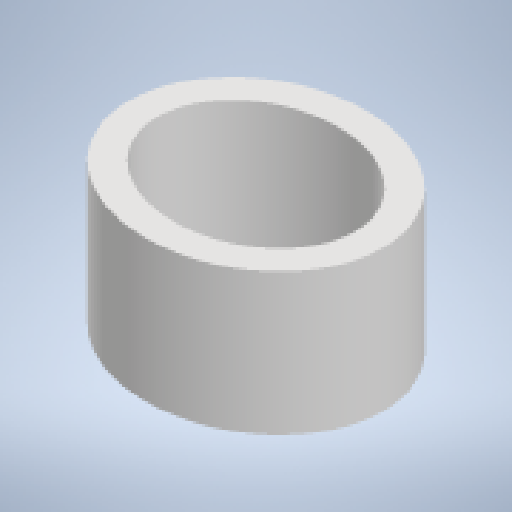
# Autodesk Inventor part: RING
Saved by Autodesk Inventor 2025.3 (Build 293356000, 356)
## iProperties
Created: 2025-05-29
Part Number: RING
Material: Generic
Document SubType Name: Modeling
Designer: Yuhsuan Chen
Density: 1 g/cm^3
Appearance: Default
Author: Yuhsuan Chen
Autodesk Inventor part; units mm, degrees
ref_plane "YZ Plane" through (0, 0, 0) normal (1, 0, 0) x (0, 1, 0)
ref_plane "XZ Plane" through (0, 0, 0) normal (0, 1, 0) x (-1, 0, 0)
ref_plane "XY Plane" through (0, 0, 0) normal (0, 0, 1) x (1, 0, 0)
sketch "Sketch1" plane through (0, 0, 0) normal (0, 1, 0) x (-1, 0, 0)
  ellipse E0 centre (0, 0) end of major axis (0, 3.9) minor radius 4.5
  ellipse E1 centre (0, 0) end of major axis (0, 2.9) minor radius 3.5
  dimension "d4" = 3.9
  dimension "d5" = 4.5
  constraints: 4 other
extrude "Extrusion1" add sketch "Sketch1" along normal blind 4.5
body "Solid1"
